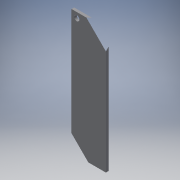
# Autodesk Inventor part: kiban
Saved by Autodesk Inventor 2016 (Build 200138000, 138)
## iProperties
Created: 2017-06-12
Part Number: kiban
Material: 一般
Document SubType Name: Modeling
Designer: B4_Ohno
Density: 1 g/cm^3
Appearance: 既定
Author: B4_Ohno
Autodesk Inventor part; units mm, degrees
ref_plane "YZ Plane" through (0, 0, 0) normal (1, 0, 0) x (0, 1, 0)
ref_plane "XZ Plane" through (0, 0, 0) normal (0, 1, 0) x (-1, 0, 0)
ref_plane "XY Plane" through (0, 0, 0) normal (0, 0, 1) x (1, 0, 0)
sketch "スケッチ1" plane through (0, 0, 0) normal (0, 1, 0) x (-1, 0, 0)
  line L0 (6.5, 23.5) -> (-6.5, 23.5)
  line L1 (-6.5, 23.5) -> (-6.5, -23.5)
  line L2 (-6.5, -23.5) -> (6.5, -23.5)
  line L3 (6.5, -23.5) -> (6.5, 23.5)
  line L4 (6.5, 23.5) -> (-6.5, -23.5) construction
  line L5 (-6.5, 23.5) -> (6.5, -23.5) construction
  point P0 (0, 0)
  dimension "d0" = 13
  dimension "d1" = 47
  constraints: 12 end point, 2 midpoint, 2 parallel, 1 horizontal, 1 perpendicular
  measures "d0" distance of L2.end L1.end
  measures "d1" distance of L1.end L0.end
extrude "押し出し1" add sketch "スケッチ1" against normal blind 1
sketch "スケッチ2" plane through (0, 0, 0) normal (0, 1, 0) x (1, 0, 0)
  circle A0 centre (-4.5, 21.5) radius 1
  line L0 (6.5, -23.5) -> (6.5, 23.5) projected
  line L1 (6.5, 23.5) -> (-6.5, 23.5) projected
  circle A1 centre (-4.5, -21.5) radius 1
  line L2 (-6.5, -23.5) -> (6.5, -23.5) projected
  point P0 (0, 0)
  dimension "d4" = 2
  dimension "d5" = 11
  dimension "d6" = 2
  dimension "d7" = 2
  dimension "d8" = 11
  dimension "d9" = 2
  constraints: 2 centre point
  measures "d4" diameter of A0
  measures "d5" distance from line of L0 A0.centre
  measures "d6" distance from line of L1 A0.centre
  measures "d7" diameter of A1
  measures "d8" distance from line of L0 A1.centre
  measures "d9" distance from line of L2 A1.centre
extrude "押し出し2" cut sketch "スケッチ2" against normal blind 1
equation "\"d7\" = d4"
equation "\"d8\" = d5"
equation "\"d9\" = d6"
